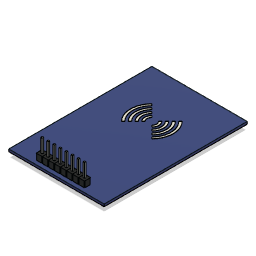
RFIDReader (Autodesk Fusion 360 design; units mm, degrees)
Autodesk Fusion 360 part; units mm, degrees
note: some values were not read from the file. Set by a fixed rule: which sketch regions a step uses.
sketch "Skizze1" plane through (0, 0, 0) normal (0, 1, 0) x (1, 0, 0)
  line L0 (0, 0) -> (40, 0)
  line L1 (40, 0) -> (40, -60)
  line L2 (40, -60) -> (0, -60)
  line L3 (0, -60) -> (0, 0)
  dimension "d1" = 40
  dimension "d2" = 60
  constraint horizontal L0
  constraint vertical L1
  constraint horizontal L2
  constraint vertical L3
  constraint coincident L0.start L3.end
  measures "d1" distance of L0.start L0.end
  measures "d2" distance of L0.start L2.end
extrude "Extrusion1" add sketch "Skizze1" along normal blind 1 makes body 1
sketch "Skizze2" plane through (0, 1, 0) normal (0, 1, 0) x (-1, 0, 0)
  line L0 (0, 60) -> (-40, 60)
  line L1 (-40, 60) -> (-40, 0)
  line L2 (-40, 0) -> (0, 0)
  line L3 (0, 0) -> (0, 60)
sketch "Skizze1 (2)" plane through (0, 0, 0) normal (0, 1, 0) x (1, 0, 0) in component "PinleistenMale v6"
  line L0 (1.27, 1.27) -> (-1.27, 1.27)
  line L1 (-1.27, 1.27) -> (-1.27, -1.27)
  line L2 (-1.27, -1.27) -> (1.27, -1.27)
  line L3 (1.27, -1.27) -> (1.27, 1.27)
  line L4 (1.27, 1.27) -> (-1.27, -1.27) construction
  line L5 (-1.27, 1.27) -> (1.27, -1.27) construction
  line L6 (0.3, -0.3) -> (-0.3, -0.3)
  line L7 (-0.3, -0.3) -> (-0.3, 0.3)
  line L8 (-0.3, 0.3) -> (0.3, 0.3)
  line L9 (0.3, 0.3) -> (0.3, -0.3)
  line L10 (0.3, -0.3) -> (-0.3, 0.3) construction
  line L11 (-0.3, -0.3) -> (0.3, 0.3) construction
  dimension "d2_1" = 2.54
  dimension "d3_1" = 2.54
  dimension "d4_1" = 0.6
  dimension "d5" = 0.6
  constraint perpendicular L0 L1
  constraint parallel L0 L2
  constraint parallel L1 L3
  constraint horizontal L0
  constraint coincident L4 origin
  constraint coincident L5 origin
  constraint perpendicular L6 L7
  constraint parallel L6 L8
  constraint parallel L7 L9
  constraint horizontal L6
  constraint coincident L10 origin
  constraint coincident L11 origin
  measures "d2_1" distance of L1.end L2.end
  measures "d3_1" distance of L0.end L1.end
  measures "d4_1" distance of L7.end L8.end
  measures "d5" distance of L6.end L7.end
extrude "Extrusion1'" add sketch "Skizze1 (2)" along normal blind 2.5 separate body makes body 2 in component "PinleistenMale v6"
fillet "Abrundung1" radius 0.2 4 edges at (-1.27, 1.25, 1.27) (1.27, 1.25, 1.27) (1.27, 1.25, -1.27) (-1.27, 1.25, -1.27) on bodies 2 in component "PinleistenMale v6"
extrude "Extrusion2" add sketch "Skizze1 (2)" along normal blind -3 and the other way blind -8.25 contours L6 L7 L8 L9 bodies 2 in component "PinleistenMale v6"
pattern_linear "R-Anordnung1" count 8 spacing 2.54 along (1, 0, 0) of bodies 2 makes body 3 at (1.5933, 2.5, -0.1) makes body 4 at (4.1333, 2.5, -0.1) makes body 5 at (6.6733, 2.5, -0.1) makes body 6 at (10.26, 2.5, 0.9467) makes body 7 at (12.8, 2.5, 0.9467) makes body 8 at (16.1867, 2.5, 0.1) makes body 9 at (17.88, 2.5, 0.9467) in component "PinleistenMale v6"
sketch "Skizze3" plane through (20, 1, 30) normal (0, 1, 0) x (-1, 0, 0)
  circle A0 centre (0, -10) radius 2
  circle A1 centre (0, -10) radius 3
  circle A2 centre (0, -10) radius 4
  circle A3 centre (0, -10) radius 5
  circle A4 centre (0, -10) radius 6
  circle A5 centre (0, -10) radius 7
  circle A6 centre (0, -10) radius 8
  circle A7 centre (0, -10) radius 9
  line L0 (-20, -30) -> (20, -30)
  line L1 (20, -30) -> (20, 30)
  circle A8 centre (0, -10) radius 10
  line L2 (-20, -30) -> (20, 10)
  line L3 (20, 30) -> (-20, 30)
  line L4 (-20, 30) -> (-20, -30)
  line L5 (-20, -30) -> (20, -30)
  line L6 (20, -30) -> (20, 30)
  line L7 (20, -30) -> (-20, 10)
  dimension "d13" = 4
  dimension "d14" = 6
  dimension "d20" = 8
  dimension "d21" = 10
  dimension "d22" = 12
  dimension "d23" = 14
  dimension "d24" = 16
  dimension "d25" = 18
  dimension "d26" = 20
  dimension "d27" = 20
  dimension "d28" = 20
  constraint concentric A0 A1
  constraint concentric A1 A2
  constraint concentric A2 A3
  constraint concentric A3 A4
  constraint concentric A2 A5
  constraint concentric A5 A6
  constraint concentric A4 A7
  constraint concentric A6 A8
  constraint coincident L0.start L2.start
  constraint coincident L1 L2.end
  constraint coincident A0.centre L2
  constraint coincident L0.end L1.start
  constraint coincident L4 L7.end
  constraint coincident A0.centre L7
  measures "d13" diameter of A0
  measures "d14" diameter of A1
  measures "d20" diameter of A2
  measures "d21" diameter of A3
  measures "d22" diameter of A4
  measures "d23" diameter of A5
  measures "d24" diameter of A6
  measures "d25" diameter of A7
  measures "d26" distance of A0.centre L0
  measures "d27" distance of A0.centre L1
  measures "d28" diameter of A8
extrude "Extrusion2'" add sketch "Skizze3" along normal blind 0.1 contours A0 A1 L2 L7 | A0 A1 L2 L7 | A2 A3 L2 L7 | A2 A3 L2 L7 | A4 A5 L2 L7 | A4 A5 L2 L7 | A6 A7 L2 L7 | A6 A7 L2 L7 picked at (2.6524, -10.2175) picked at (-1.9791, -11.7778) picked at (4.641, -10.3916) picked at (-3.5801, -12.9763) picked at (5.0878, -14.2879) picked at (-5.6712, -6.5249) picked at (6.387, -4.1668) picked at (-6.6577, -4.4828) bodies 1
component "PinleistenMale v6" placed x (1, 0, 0) y (0, 1, 0) z (0, 0, 1) at (11, 1, 57)
equation "p = 2.54 mm"
equation "d2_1 = p"
equation "d3_1 = p"
equation "Anzahl_x = 8"
equation "Anzahl_y = 1"
equation "d15 = Anzahl_x"
equation "d16 = Anzahl_y"
equation "d17 = p"
equation "d18 = p"
